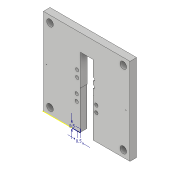
# Autodesk Inventor part: top STAND PLATE FOR STORSGE SYSTEM
Saved by Autodesk Inventor 2019 (Build 230136000, 136)
## iProperties
Created: 2019-10-14
Part Number: top STAND PLATE FOR STORSGE SYSTEM
Material: Generic
Document SubType Name: Modeling
Designer: Admin
Density: 1 g/cm^3
Appearance: Default
Author: Admin
Autodesk Inventor part; units mm, degrees
ref_plane "YZ Plane" through (0, 0, 0) normal (1, 0, 0) x (0, 1, 0)
ref_plane "XZ Plane" through (0, 0, 0) normal (0, 1, 0) x (-1, 0, 0)
ref_plane "XY Plane" through (0, 0, 0) normal (0, 0, 1) x (1, 0, 0)
sketch "Sketch1" plane through (0, 0, 0) normal (0, 0, 1) x (1, 0, 0)
  line L0 (0, 0) -> (130, 0)
  line L1 (130, 0) -> (130, 130)
  line L2 (130, 130) -> (0, 130)
  line L3 (0, 130) -> (0, 0)
  dimension "d0" = 130
  dimension "d1" = 130
  constraints: 8 end point, 2 parallel, 1 horizontal, 1 perpendicular
  measures "d0" distance of L2.end L1.end
  measures "d1" distance of L1.end L0.end
extrude "Extrusion1" add sketch "Sketch1" along normal blind 10
sketch "Sketch2" plane through (0, 0, 10) normal (0, 0, 1) x (1, 0, 0)
  line L0 (0, 0) -> (130, 0) projected
  line L1 (0, 0) -> (10, 0)
  line L2 (10, 0) -> (10, 110)
  line L3 (10, 110) -> (10, 120)
  line L4 (10, 120) -> (120, 120)
  line L5 (120, 120) -> (120, 10)
  line L6 (120, 10) -> (10, 10)
  circle A0 centre (10, 120) radius 5
  circle A1 centre (120, 120) radius 5
  circle A2 centre (10, 10) radius 5
  circle A3 centre (120, 10) radius 5
  dimension "d4" = 10
  dimension "d5" = 110
  dimension "d6" = 10
  dimension "d7" = 110
  dimension "d8" = 110
  dimension "d9" = 110
  dimension "d10" = 10
  dimension "d11" = 10
  dimension "d12" = 10
  dimension "d13" = 10
  constraints: 12 end point, 4 centre point, 4 coincident, 3 perpendicular, 3 point on line
  measures "d4" distance of L0.start L1.end
  measures "d5" distance of L1.end L2.end
  measures "d6" distance of L2.end L3.end
  measures "d7" distance of L3.end L4.end
  measures "d8" distance of L4.end L5.end
  measures "d9" distance of L5.end L6.end
  measures "d10" diameter of A0
  measures "d11" diameter of A1
  measures "d12" diameter of A2
  measures "d13" diameter of A3
extrude "Extrusion2" cut sketch "Sketch2" against normal through all contours A2 L2 | L2 L6 A2 | L2 A2 L6 | A3 L5 L6 | L6 L5 A3 | A0 L4 L3 | L3 L4 A0 | A1 L4 L5 | L5 L4 A1
sketch "Sketch3" plane through (0, 0, 10) normal (0, 0, 1) x (1, 0, 0)
  line L0 (0, 0) -> (130, 0) projected
  line L1 (68.2625, 0) -> (63.2625, 0)
  line L2 (63.2625, 0) -> (63.2625, 5)
  circle A0 centre (63.2625, 5) radius 0.05
  dimension "d16" = 5
  dimension "d17" = 5
  dimension "d18" = 0.1
  constraints: 4 end point, 2 point on line, 1 centre point, 1 coincident, 1 perpendicular
  measures "d16" distance of L1.start L1.end
  measures "d17" distance of L1.end L2.end
  measures "d18" diameter of A0
extrude "Extrusion3" cut sketch "Sketch3" along normal through all both and the other way through all
sketch "Sketch4" plane through (0, 0, 10) normal (0, 0, 1) x (1, 0, 0)
  line L0 (63.5, 131.7625) -> (63.5, 126.7625)
  circle A0 centre (63.5, 126.7625) radius 0.05
  point P0 (0, 0)
  dimension "d21" = 5
  dimension "d22" = 0.1
  constraints: 2 end point, 1 centre point, 1 coincident, 1 vertical
  measures "d21" distance of L0.start L0.end
  measures "d22" diameter of A0
extrude "Extrusion4" cut sketch "Sketch4" against normal blind 10
sketch "Sketch5" plane through (0, 0, 10) normal (0, 0, 1) x (1, 0, 0)
  line L0 (0, 63.5) -> (5, 63.5)
  line L1 (5, 63.5) -> (123.825, 63.5)
  circle A0 centre (5, 63.5) radius 0.5
  circle A1 centre (123.825, 63.5) radius 0.5
  point P0 (0, 0)
  dimension "d25" = 5
  dimension "d26" = 1
  dimension "d27" = 1
  constraints: 4 end point, 2 centre point, 2 coincident, 1 horizontal, 1 point on line
  measures "d25" distance of L0.start L0.end
  measures "d26" diameter of A0
  measures "d27" diameter of A1
extrude "Extrusion5" cut sketch "Sketch5" against normal through all
sketch "Sketch6" plane through (0, 0, 10) normal (0, 0, 1) x (1, 0, 0)
  point P0 (0, 0)
sketch "Sketch7" plane through (0, 0, 10) normal (0, 0, 1) x (1, 0, 0)
  line L0 (0, 0) -> (55, 0)
  line L1 (0, 0) -> (130, 0) projected
  line L2 (55, 0) -> (75, 0)
  line L3 (75, 0) -> (130, 0)
  line L4 (55, 0) -> (75, 0)
  line L5 (75, 0) -> (75, 58)
  line L6 (75, 58) -> (55, 58)
  line L7 (55, 58) -> (55, 0)
  dimension "d30" = 55
  dimension "d31" = 20
  dimension "d32" = 55
  dimension "d33" = 20
  dimension "d34" = 58
  constraints: 14 end point, 3 point on line, 2 parallel, 1 horizontal, 1 perpendicular
  measures "d30" distance of L0.start L0.end
  measures "d31" distance of L0.end L2.end
  measures "d32" distance of L2.end L3.end
  measures "d33" distance of L6.end L5.end
  measures "d34" distance of L5.end L4.end
extrude "Extrusion6" cut sketch "Sketch7" against normal blind 10
sketch "Sketch8" plane through (0, 0, 10) normal (0, 0, 1) x (1, 0, 0)
  line L0 (74.6125, 0) -> (79.6125, 0)
  line L1 (79.6125, 0) -> (79.6125, 38)
  line L2 (79.6125, 38) -> (79.6125, 48)
  line L3 (55, 58) -> (55, 0) projected
  line L4 (55, 0) -> (50, 0)
  line L5 (0, 0) -> (55, 0) projected
  line L6 (50, 0) -> (50, 38)
  line L7 (50, 38) -> (50, 48)
  circle A0 centre (79.6125, 48) radius 2.5
  circle A1 centre (79.6125, 38) radius 2.5
  circle A2 centre (50, 48) radius 2.5
  circle A3 centre (50, 38) radius 2.5
  dimension "d37" = 5
  dimension "d38" = 38
  dimension "d39" = 10
  dimension "d40" = 5
  dimension "d41" = 38
  dimension "d42" = 10
  dimension "d43" = 5
  dimension "d44" = 5
  dimension "d45" = 5
  dimension "d46" = 5
  constraints: 12 end point, 4 centre point, 4 coincident, 3 point on line, 2 perpendicular, 1 horizontal
  measures "d37" distance of L0.start L0.end
  measures "d38" distance of L0.end L1.end
  measures "d39" distance of L1.end L2.end
  measures "d40" distance of L3.end L4.end
  measures "d41" distance of L4.end L6.end
  measures "d42" distance of L6.end L7.end
  measures "d43" diameter of A0
  measures "d44" diameter of A1
  measures "d45" diameter of A2
  measures "d46" diameter of A3
extrude "Extrusion7" cut sketch "Sketch8" against normal through all
sketch "Sketch9" plane through (0, 0, 10) normal (0, 0, 1) x (1, 0, 0)
  line L0 (55.5625, 57.15) -> (74.6125, 57.15)
  line L1 (74.6125, 57.15) -> (74.6125, 104.775)
  line L2 (74.6125, 104.775) -> (55.5625, 104.775)
  line L3 (55.5625, 104.775) -> (55.5625, 57.15)
  point P0 (0, 0)
  constraints: 8 end point, 2 parallel, 1 horizontal, 1 perpendicular
extrude "Extrusion8" cut sketch "Sketch9" against normal blind 10
sketch "Sketch10" plane through (0, 0, 10) normal (0, 0, 1) x (1, 0, 0)
  line L0 (0, 0) -> (55, 0) projected
  line L1 (55, 0) -> (55, 5)
  line L2 (55, 0) -> (42.8625, 0)
  dimension "d51" = 5
  constraints: 4 end point, 1 perpendicular, 1 point on line
  measures "d51" distance of L0.end L1.end
sketch "Sketch11" plane through (0, 0, 10) normal (0, 0, 1) x (1, 0, 0)
  line L0 (55.5625, 0) -> (50.5625, 0)
  line L1 (0, 0) -> (55, 0) projected
  dimension "d52" = 5
  constraints: 2 end point, 1 point on line
  measures "d52" distance of L0.start L0.end
sketch "Sketch12" plane through (0, 0, 10) normal (0, 0, 1) x (1, 0, 0)
  line L0 (75, 58) -> (75, 0) projected
  line L1 (75, 0) -> (80, 0)
  line L2 (75, 0) -> (130, 0) projected
  line L3 (80, 0) -> (80, 85.725)
  line L4 (80, 85.725) -> (80, 100.0125)
  line L5 (50.8, 0) -> (50.8, 69.4562)
  line L6 (55, 0) -> (55, 58) projected
  line L7 (50.8, 69.4562) -> (50.8, 79.4562)
  line L8 (50.8, 79.4562) -> (80, 79.4562)
  circle A0 centre (50.8, 79.4562) radius 2.5
  circle A1 centre (50.8, 69.4562) radius 2.5
  line L9 (50.8, 69.4562) -> (80, 69.4562)
  line L10 (80, 79.4562) -> (82.5, 79.4562)
  line L11 (82.5, 79.4562) -> (77.5, 79.4562)
  line L12 (77.5, 79.4562) -> (77.5, 69.4562)
  circle A2 centre (74.6125, 79.4562) radius 2.5
  circle A3 centre (74.6125, 69.4562) radius 2.5
  point P0 (0, 0)
  dimension "d53" = 5
  dimension "d54" = 10
  dimension "d55" = 5
  dimension "d56" = 5
  dimension "d61" = 2.5
  dimension "d62" = 5
  dimension "d64" = 5
  dimension "d65" = 5
  constraints: 20 end point, 9 point on line, 4 centre point, 3 perpendicular, 2 coincident, 1 parallel, 1 vertical
  measures "d53" distance of L0.end L1.end
  measures "d54" distance of L5.end L7.end
  measures "d55" diameter of A0
  measures "d56" diameter of A1
  measures "d61" distance of L8.end L10.end
  measures "d62" distance of L10.end L11.end
  measures "d64" diameter of A2
  measures "d65" diameter of A3
extrude "Extrusion9" cut sketch "Sketch12" against normal blind 10 contours A3 L9 | L9 A3 | A2 L8 | L8 A2 | L9 L7 A1 | A1 L5 L9 | A0 L7 L8 | L8 L7 A0 | L7 L5 A1
body "Solid1"
